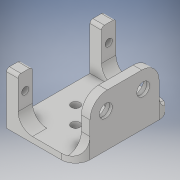
# Autodesk Inventor part: bracket
Saved by Autodesk Inventor 2019 (Build 230136000, 136)
## iProperties
Created: 2019-01-20
Part Number: bracket
Material: Generic
Document SubType Name: Modeling
Designer: Daniel
Density: 1 g/cm^3
Appearance: Default
Author: Daniel
Autodesk Inventor part; units mm, degrees
ref_plane "YZ Plane" through (0, 0, 0) normal (1, 0, 0) x (0, 1, 0)
ref_plane "XZ Plane" through (0, 0, 0) normal (0, 1, 0) x (-1, 0, 0)
ref_plane "XY Plane" through (0, 0, 0) normal (0, 0, 1) x (1, 0, 0)
sketch "Sketch1" plane through (0, 0, 0) normal (0, 1, 0) x (-1, 0, 0)
  line L0 (15.4, 0) -> (-15.4, 0) projected
  line L1 (0, -23.8) -> (0, 23.8) projected
  line L2 (11, 17) -> (-11, 17)
  line L3 (-11, 17) -> (-11, -17)
  line L4 (-11, -17) -> (11, -17)
  line L5 (11, -17) -> (11, 17)
  point P0 (0, 0)
  dimension "d0" = 22
  dimension "d1" = 34
  constraints: 8 end point, 2 parallel, 1 horizontal, 1 perpendicular, 2 other
  measures "d0" distance between parallel lines of L3 L5
  measures "d1" distance between parallel lines of L4 L2
extrude "Extrusion1" add sketch "Sketch1" along normal blind 18
sketch "Sketch2" plane through (0, 18, 0) normal (0, 1, 0) x (1, 0, 0)
  line L0 (-11, -12) -> (8, -12)
  line L1 (8, -12) -> (8, 12)
  line L2 (8, 12) -> (-11, 12)
  line L3 (-11, 12) -> (-11, -12)
  line L4 (-11, -17) -> (11, -17) projected
  line L5 (11, -17) -> (11, 17) projected
  line L6 (11, 17) -> (-11, 17) projected
  line L7 (-11, 17) -> (-11, -17) projected
  line L8 (-15.4, 0) -> (15.4, 0) projected
  point P0 (0, 0)
  dimension "d5" = 24
  dimension "d6" = 3
  constraints: 8 end point, 2 parallel, 1 collinear, 1 horizontal, 1 perpendicular, 1 other
  measures "d5" distance between parallel lines of L2 L0
  measures "d6" distance between parallel lines of L5 L1
extrude "Extrusion2" cut sketch "Sketch2" against normal blind 16 contours L3 L8 L1 L0 | L3 L2 L1 L8
sketch "Sketch3" plane through (-11, 0, 17) normal (0, 0, 1) x (1, 0, 0)
  line L0 (4, 18) -> (19, 18)
  line L1 (19, 18) -> (19, 2)
  line L2 (19, 2) -> (4, 2)
  line L3 (4, 2) -> (4, 18)
  line L4 (0, 18) -> (22, 18) projected
  line L5 (0, 0) -> (0, 18) projected
  line L6 (22, 0) -> (22, 18) projected
  line L7 (0, 0) -> (22, 0) projected
  point P0 (11, 0)
  dimension "d9" = 4
  dimension "d10" = 3
  dimension "d11" = 2
  constraints: 8 end point, 2 parallel, 1 collinear, 1 horizontal, 1 perpendicular
  measures "d9" distance between parallel lines of L5 L3
  measures "d10" distance between parallel lines of L6 L1
  measures "d11" distance between parallel lines of L7 L2
extrude "Extrusion3" cut sketch "Sketch3" against normal through all contours L0 L1 L2 L3
sketch "Sketch6" plane through (0, 2, 0) normal (0, 1, 0) x (1, 0, 0)
  line L0 (-11, 12) -> (-7, 12) projected
  line L1 (-11, -12) -> (-11, 12) projected
  line L2 (-7, -12) -> (-11, -12) projected
  line L3 (-7, -17) -> (-7, -12) projected
  line L4 (8, -17) -> (-7, -17) projected
  line L5 (-7, 17) -> (8, 17) projected
  line L6 (-7, 12) -> (-7, 17) projected
  line L7 (-15.4, 0) -> (15.4, 0) projected
  line L8 (0, 23.8) -> (0, -23.8) projected
  line L9 (8, -17) -> (8, 17) projected
  point P0 (0, 0)
  point P1 (0, 0)
  point P2 (0, 6)
  point P3 (0, -6)
  point P4 (-6, 0)
  dimension "d15" = 6
  dimension "d16" = 6
  dimension "d18" = 6
  constraints: 3 point on line, 1 coincident
  measures "d15" distance of point (0, 0) point (0, 6)
  measures "d16" distance of point (0, 0) point (-6, 0)
  measures "d18" distance of point (0, 0) point (0, -6)
hole "Hole1" at (0, 2, -6) at (0, 2, 0) at (0, 2, 6) at (-6, 2, 0) direction (0, -1, 0) diameter 3 end through all
sketch "Sketch8" plane through (11, 0, 17) normal (1, 0, 0) x (0, 0, -1)
  line L0 (0, 0) -> (34, 0) projected
  line L1 (34, 0) -> (34, 18) projected
  line L2 (0, 18) -> (34, 18) projected
  line L3 (0, 0) -> (0, 18) projected
  line L4 (29, 2) -> (29, 18) projected
  line L5 (5, 18) -> (5, 2) projected
  line L6 (29, 2) -> (5, 2) projected
  point P0 (17, 0)
  point P1 (0, 2)
  point P2 (34, 2)
  point P3 (23.5, 12)
  point P4 (10.5, 12)
  dimension "d28" = 5.5
  dimension "d29" = 5.5
  dimension "d30" = 6
  dimension "d31" = 6
  measures "d28" distance from line of L4 point (23.5, 12)
  measures "d29" distance from line of L5 point (10.5, 12)
  measures "d30" distance from line of L2 point (10.5, 12)
  measures "d31" distance from line of L2 point (23.5, 12)
hole "Hole2" at (11, 12, -6.5) at (11, 12, 6.5) direction (-1, 0, 0) diameter 4.5 end through all
sketch "Sketch12" plane through (0, 18, 0) normal (0, 1, 0) x (1, 0, 0)
  line L0 (8, 17) -> (8, -17) projected
  line L1 (8, -17) -> (11, -17) projected
  line L2 (11, -17) -> (11, 17) projected
  line L3 (11, 17) -> (8, 17) projected
  line L4 (8, -17) -> (11, -17)
  line L5 (11, -17) -> (11, -12)
  line L6 (11, -12) -> (8, -12)
  line L7 (8, -12) -> (8, -17)
  line L8 (8, 17) -> (11, 17)
  line L9 (11, 17) -> (11, 12)
  line L10 (11, 12) -> (8, 12)
  line L11 (8, 12) -> (8, 17)
  line L12 (-7, -17) -> (-7, -12) projected
  line L13 (-7, -12) -> (-11, -12) projected
  line L14 (-11, -12) -> (-11, -17) projected
  line L15 (-11, -17) -> (-7, -17) projected
  line L16 (-7, 12) -> (-7, 17) projected
  line L17 (-7, 17) -> (-11, 17) projected
  line L18 (-11, 17) -> (-11, 12) projected
  line L19 (-11, 12) -> (-7, 12) projected
  point P0 (0, 0)
  constraints: 16 end point, 8 collinear, 4 parallel, 2 horizontal, 2 perpendicular
extrude "Extrusion5" cut sketch "Sketch12" against normal blind 16 contours L3 L2 L10 L0 | L6 L2 L1 L0
sketch "Sketch17" plane through (-11, 0, -17) normal (-1, 0, 0) x (0, 0, 1)
  line L0 (29, 18) -> (29, 2) projected
  line L1 (29, 2) -> (5, 2) projected
  line L2 (5, 2) -> (5, 18) projected
  line L3 (0, 18) -> (5, 18) projected
  line L4 (0, 0) -> (0, 18) projected
  line L5 (0, 0) -> (34, 0) projected
  line L6 (34, 0) -> (34, 18) projected
  line L7 (29, 18) -> (34, 18) projected
  line L8 (34, 0) -> (0, 0) projected
  line L9 (29, 18) -> (29, 2) projected
  line L10 (34, 0) -> (29, 0)
  line L11 (29, 0) -> (29, 18)
  line L12 (29, 18) -> (34, 18)
  line L13 (34, 18) -> (34, 0)
  line L14 (0, 18) -> (5, 18) projected
  line L15 (0, 0) -> (5, 0)
  line L16 (5, 0) -> (5, 18)
  line L17 (5, 18) -> (0, 18)
  line L18 (0, 18) -> (0, 0)
  line L19 (0, 2) -> (5, 2) projected
  line L20 (34, 0) -> (0, 0)
  line L21 (0, 0) -> (0, 2)
  line L22 (0, 2) -> (34, 2)
  line L23 (34, 2) -> (34, 0)
  point P0 (17, 0)
  constraints: 24 end point, 6 parallel, 3 horizontal, 3 perpendicular
extrude "Extrusion6" add sketch "Sketch17" along normal blind 2
sketch "Sketch19" plane through (8, 18, -12) normal (-1, 0, 0) x (0, 0, 1)
  circle A0 centre (18.5, -6) radius 2.25 projected
  circle A1 centre (5.5, -6) radius 2.25 projected
  line L0 (24, -16) -> (24, 0) projected
  line L1 (0, 0) -> (24, 0) projected
  line L2 (0, 0) -> (0, -16) projected
  line L3 (24, -16) -> (0, -16) projected
  point P0 (12, -18)
  constraints: 2 coincident
hole "Hole4" at (8, 12, 6.5) at (8, 12, -6.5) direction (1, 0, 0) diameter 6.5 depth 2
fillet "Fillet9" radius 6 2 edges at (9.5, 18, -12) (9.5, 18, 12)
fillet "Fillet10" radius 5 4 edges at (9.5, 2, 12) (9.5, 2, -12) (11, 1, 17) (11, 1, -17)
sketch "Sketch20" plane through (-13, 0, -17) normal (-1, 0, 0) x (0, 0, 1)
  line L0 (0, 0) -> (34, 0) projected
  line L1 (34, 0) -> (34, 18) projected
  line L2 (34, 18) -> (29, 18) projected
  line L3 (29, 18) -> (29, 2) projected
  line L4 (29, 2) -> (5, 2) projected
  line L5 (5, 2) -> (5, 18) projected
  line L6 (5, 18) -> (0, 18) projected
  line L7 (0, 18) -> (0, 0) projected
  point P0 (17, 0)
  point P1 (2.5, 12)
  point P2 (31.5, 12)
  dimension "d85" = 6
  dimension "d86" = 2.5
  dimension "d87" = 2.5
  dimension "d88" = 6
  measures "d85" distance from line of L6 point (2.5, 12)
  measures "d86" distance from line of L5 point (2.5, 12)
  measures "d87" distance from line of L3 point (31.5, 12)
  measures "d88" distance from line of L2 point (31.5, 12)
hole "Hole5" at (-13, 12, -14.5) at (-13, 12, 14.5) direction (1, 0, 0) diameter 2.5 end through all
sketch "Sketch21" plane through (-7, 2, 17) normal (0, 0, 1) x (1, 0, 0)
  line L0 (-2, 16) -> (0, 16)
  line L1 (0, 16) -> (0, 0)
  line L2 (0, 0) -> (-2, 0)
  line L3 (-2, 0) -> (-2, 16)
  line L4 (13, 0) -> (13, -2) projected
  line L5 (13, 0) -> (0, 0) projected
  line L6 (0, 0) -> (0, 16) projected
  line L7 (0, 16) -> (-6, 16) projected
  line L8 (-6, -2) -> (-6, 16) projected
  line L9 (-6, -2) -> (13, -2) projected
  line L10 (13, 0) -> (0, 0) projected
  line L11 (0, 16) -> (-6, 16) projected
  line L12 (0, 0) -> (0, 16) projected
  point P0 (7, -2)
  dimension "d96" = 4
  constraints: 8 end point, 3 collinear, 2 parallel, 1 horizontal, 1 perpendicular
  measures "d96" distance between parallel lines of L8 L3
extrude "Extrusion7" cut sketch "Sketch21" against normal through all contours L0 L1 L2 L3
fillet "Fillet11" radius 5 2 edges at (-9, 2, 14.5) (-9, 2, -14.5)
fillet "Fillet12" radius 1 4 edges at (-11, 18, 17) (-11, 18, 12) (-11, 18, -12) (-11, 18, -17)
body "Solid1"
